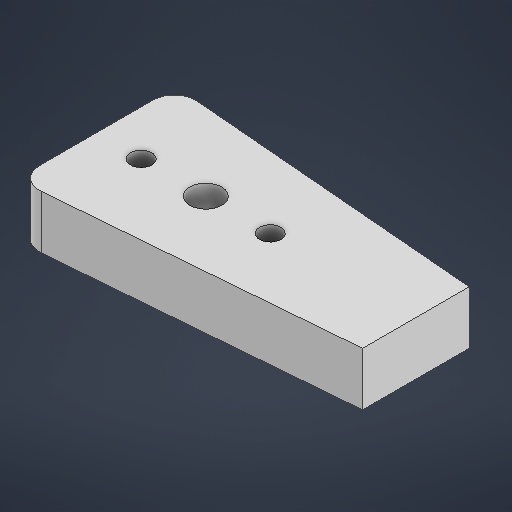
# Autodesk Inventor part: хуйня резня
Saved by Autodesk Inventor 2026.2 (Build 302298000, 298)
## iProperties
Created: 2026-01-16
Part Number: хуйня резня
Material: Типовые
Document SubType Name: Modeling
Designer: Phantom
Density: 1 g/cm^3
Appearance: По умолчанию
Author: Phantom
Autodesk Inventor part; units mm, degrees
ref_plane "YZ Plane" through (0, 0, 0) normal (1, 0, 0) x (0, 1, 0)
ref_plane "XZ Plane" through (0, 0, 0) normal (0, 1, 0) x (-1, 0, 0)
ref_plane "XY Plane" through (0, 0, 0) normal (0, 0, 1) x (1, 0, 0)
sketch "Эскиз1" plane through (0, 0, 0) normal (0, 1, 0) x (-1, 0, 0)
  line L0 (35, 15.6528) -> (35, -5.6528)
  line L1 (-25, -5) -> (-25, 15)
  line L2 (30.6678, 19.639) -> (-25, 15)
  line L3 (30.6678, -9.639) -> (-25, -5)
  circle A0 centre (2.3404, 5) radius 2
  circle A1 centre (14.4404, 5) radius 3
  circle A2 centre (26.5404, 5) radius 2
  arc A3 (35, 15.6528) -> (30.6678, 19.639) centre (31, 15.6528) ccw
  arc A4 (30.6678, -9.639) -> (35, -5.6528) centre (31, -5.6528) ccw
  point P0 (0, 0)
  point P1 (35, -10)
  point P2 (35, 20)
  point P3 (12.9676, -25.8489)
  dimension "d0" = 30
  dimension "d4" = 60
  dimension "d6" = 15
  dimension "d8" = 4
  constraints: 8 end point, 5 centre point, 4 point on circle, 4 point on line, 4 tangent, 1 equal radius, 1 parallel
  measures "d0" distance of point (35, 20) point (35, -10)
  measures "d4" distance between parallel lines of L0 L1
  measures "d6" vertical distance of L1.end point (0, 0)
  measures "d8" radius of A3
extrude "Выдавливание1" add sketch "Эскиз1" along normal blind 10
